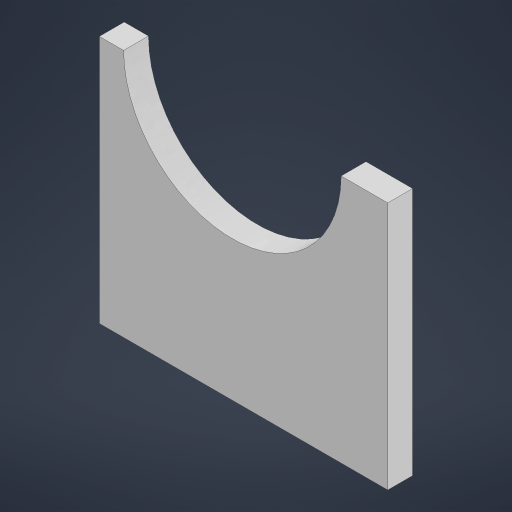
# Autodesk Inventor part: Weldedsupportpart1
Saved by Autodesk Inventor 2023 (Build 270158000, 158)
## iProperties
Created: 2022-09-04
Part Number: Weldedsupportpart1
Material: Generic
Document SubType Name: Modeling
Designer: Mike
Density: 1 g/cm^3
Appearance: Default
Author: Mike
Autodesk Inventor part; units mm, degrees
ref_plane "YZ Plane" through (0, 0, 0) normal (1, 0, 0) x (0, 1, 0)
ref_plane "XZ Plane" through (0, 0, 0) normal (0, 1, 0) x (-1, 0, 0)
ref_plane "XY Plane" through (0, 0, 0) normal (0, 0, 1) x (1, 0, 0)
sketch "Sketch1" plane through (0, 0, 0) normal (0, 0, 1) x (1, 0, 0)
  arc A0 (-87.5, 200) -> (87.5, 200) centre (0, 200) ccw
  line L0 (87.5, 200) -> (125, 200)
  line L1 (125, 200) -> (125, 0)
  line L2 (125, 0) -> (-107, 0)
  line L3 (-107, 0) -> (-107, 200)
  line L4 (-107, 200) -> (-87.5, 200)
  point P0 (0, 0)
  dimension "d0" = 200
  dimension "d1" = 175
  dimension "d2" = 37.5
  dimension "d3" = 232
  dimension "d4" = 125
  dimension "d5" = 200
  constraints: 10 end point, 3 perpendicular, 2 point on circle, 2 point on line, 1 centre point, 1 horizontal, 1 vertical alignment
  measures "d0" distance of A0.centre point (0, 0)
  measures "d1" diameter of A0
  measures "d2" distance of L0.start L0.end
  measures "d3" distance of L1.end L2.end
  measures "d4" distance from line of L1 point (0, 0)
  measures "d5" distance between parallel lines of L2 L0
extrude "Extrusion1" add sketch "Sketch1" against normal blind 20
body "Solid1"
